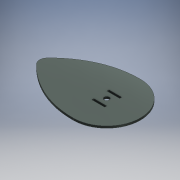
# Autodesk Inventor part: leva00
Saved by Autodesk Inventor 2016 (Build 200138000, 138)
## iProperties
Created: 2016-09-20
Part Number: leva00
Material: Madera (abedul)
Document SubType Name: Modeling
Designer: i95sa
Density: 0.55 g/cm^3
Appearance: Gris plomo - Pulido
Author: i95sa
Autodesk Inventor part; units mm, degrees
ref_plane "YZ Plane" through (0, 0, 0) normal (1, 0, 0) x (0, 1, 0)
ref_plane "XZ Plane" through (0, 0, 0) normal (0, 1, 0) x (-1, 0, 0)
ref_plane "XY Plane" through (0, 0, 0) normal (0, 0, 1) x (1, 0, 0)
sketch "Boceto1" plane through (0, 0, 0) normal (0, 0, 1) x (1, 0, 0)
  arc A0 (65, 0) -> (-65, 0) centre (0, 0) ccw
  arc A1 (-100.0299, 0) -> (-130.0299, 0) centre (-115.0299, 0) ccw
  line L0 (-134.3728, 0) -> (-134.3728, 15)
  line L1 (0.77, 64.9954) -> (0.77, 89.9954)
  line L2 (0.77, 89.9954) -> (-134.3728, 15)
  line L3 (-134.3728, 15) -> (-81.9095, 44.1137)
  arc A2 (0.77, 64.9954) -> (-81.9095, 44.1137) centre (-1.2004, -101.3252) ccw
  arc A3 (-81.9095, 44.1137) -> (-125.8146, 10.4254) centre (9.2294, -120.1197) ccw
  line L4 (5, 0) -> (65, 0)
  line L5 (-5, 0) -> (-134.3728, 0)
  arc A4 (-65, 0) -> (65, 0) centre (0, 0) ccw
  arc A5 (-130.0299, 0) -> (-100.0299, 0) centre (-115.0299, 0) ccw
  line L6 (-134.3728, 0) -> (-134.3728, -15)
  line L7 (0.77, -64.9954) -> (0.77, -89.9954)
  line L8 (0.77, -89.9954) -> (-134.3728, -15)
  line L9 (-134.3728, -15) -> (-81.9095, -44.1137)
  arc A6 (-81.9095, -44.1137) -> (0.77, -64.9954) centre (-1.2004, 101.3252) ccw
  arc A7 (-125.8146, -10.4254) -> (-81.9095, -44.1137) centre (9.2294, 120.1197) ccw
  dimension "d0" = 130
  dimension "d6" = 30
  dimension "d7" = 15
  dimension "d8" = 25
  dimension "d9" = 60
  constraints: 20 end point, 20 point on circle, 8 centre point, 6 symmetric about line, 5 point on line, 4 tangent, 2 vertical, 1 collinear, 1 horizontal, 4 other
  measures "d0" diameter of A0
  measures "d6" diameter of A1
  measures "d7" distance of L0.start L0.end
  measures "d8" distance of L1.start L1.end
  measures "d9" distance of L0.end L3.end
extrude "Extrusión2" add sketch "Boceto1" along normal blind 4 contours A4 A0 | A0 L5 A1 A3 A2 | A6 A7 A5 L5 A4 | L5 A1 | A5 L5
sketch "Boceto2" plane through (0, 0, 4) normal (0, 0, 1) x (1, 0, 0)
  line L0 (0, 0) -> (0, 12.5)
  line L1 (0, 12.5) -> (-12.5, 12.5)
  line L2 (-12.5, 12.5) -> (-12.5, 16.7)
  line L3 (-12.5, 16.7) -> (12.5, 16.7)
  line L4 (12.5, 16.7) -> (12.5, 12.5)
  line L5 (12.5, 12.5) -> (0, 12.5)
  line L6 (0, 0) -> (12.5, 0)
  line L7 (0, 0) -> (0, -12.5)
  line L8 (0, -12.5) -> (-12.5, -12.5)
  line L9 (-12.5, -12.5) -> (-12.5, -16.7)
  line L10 (-12.5, -16.7) -> (12.5, -16.7)
  line L11 (12.5, -16.7) -> (12.5, -12.5)
  line L12 (12.5, -12.5) -> (0, -12.5)
  circle A0 centre (0, 0) radius 5
  dimension "d24" = 12.5
  dimension "d25" = 12.5
  dimension "d26" = 4.2
  dimension "d27" = 25
  dimension "d28" = 10
  constraints: 26 end point, 5 perpendicular, 5 symmetric about line, 3 point on line, 1 centre point, 1 coincident, 1 parallel, 1 vertical
  measures "d24" distance of L0.start L0.end
  measures "d25" distance of L0.end L1.end
  measures "d26" distance of L1.end L2.end
  measures "d27" distance of L2.end L3.end
  measures "d28" diameter of A0
extrude "Extrusión3" cut sketch "Boceto2" against normal blind 4
